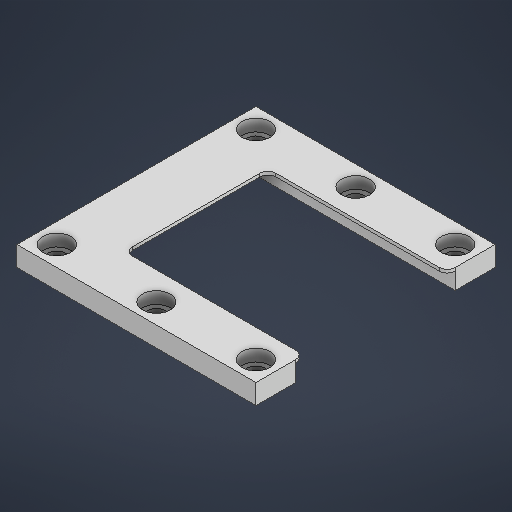
# Autodesk Inventor part: Flex Circuit Clamp V1
Saved by Autodesk Inventor 2026.2 (Build 302298010, 298A)
## iProperties
Created: 2026-05-04
Part Number: Flex Circuit Clamp V1
Material: Generic
Document SubType Name: Modeling
Designer: cfang
Density: 1 g/cm^3
Appearance: Default
Author: cfang
Autodesk Inventor part; units mm, degrees
ref_plane "YZ Plane" through (0, 0, 0) normal (1, 0, 0) x (0, 1, 0)
ref_plane "XZ Plane" through (0, 0, 0) normal (0, 1, 0) x (-1, 0, 0)
ref_plane "XY Plane" through (0, 0, 0) normal (0, 0, 1) x (1, 0, 0)
sketch "Sketch1" plane through (0, 0, 0) normal (0, 1, 0) x (-1, 0, 0)
  line L0 (-15, -15) -> (15, -15)
  line L1 (15, -15) -> (15, 15)
  line L2 (15, 15) -> (-15, 15)
  line L3 (-15, 15) -> (-15, -15)
  line L4 (-15, -15) -> (15, 15) construction
  line L5 (15, -15) -> (-15, 15) construction
  point P0 (0, 0)
  dimension "d0" = 30
  dimension "d1" = 30
  constraints: 12 end point, 2 midpoint, 2 parallel, 1 horizontal, 1 perpendicular
  measures "d0" distance of L0.end L1.end
  measures "d1" distance of L1.end L2.end
extrude "Extrusion1" add sketch "Sketch1" along normal blind 2.5
sketch "Sketch2" plane through (0, 2.5, 0) normal (0, 1, 0) x (1, 0, 0)
  line L0 (15, -15) -> (15, 15) projected
  line L1 (15, -10) -> (-10, -10)
  line L2 (-10, -10) -> (-10, 10)
  line L3 (-10, 10) -> (15, 10)
  line L4 (15, 10) -> (15, -10)
  point P0 (0, 0)
  point P1 (15, 10)
  dimension "d4" = 20
  dimension "d5" = 10
  dimension "d6" = 25
  constraints: 8 end point, 2 parallel, 1 horizontal, 1 perpendicular, 1 point on line
  measures "d4" distance of L1.end L2.end
  measures "d5" distance from line of L1 point (0, 0)
  measures "d6" distance of L1.start L1.end
extrude "Extrusion2" cut sketch "Sketch2" against normal through all
sketch "Sketch3" plane through (0, 2.5, 0) normal (0, 1, 0) x (1, 0, 0)
  line L0 (15, -10) -> (-10, -10) projected
  line L1 (-10, -10) -> (-10, 10) projected
  line L2 (-10, 10) -> (15, 10) projected
  line L3 (15, -10) -> (-10, -10)
  line L4 (-10, -10) -> (-10, -9)
  line L5 (-6.5, -9) -> (14, -9)
  line L6 (15, -10) -> (15, -10)
  line L7 (15, 10) -> (-10, 10)
  line L8 (-10, 10) -> (-10, 9)
  line L9 (-6.5, 9) -> (14, 9)
  line L10 (15, 10) -> (15, 10)
  line L11 (-10, -10) -> (-7.5, -10)
  line L12 (-7.5, -8) -> (-7.5, 8)
  line L13 (-7.5, 10) -> (-10, 10)
  line L14 (-10, 10) -> (-10, -10)
  arc A0 (15, -10) -> (14, -9) centre (14, -10) ccw
  arc A1 (-7.5, -8) -> (-6.5, -9) centre (-6.5, -8) ccw
  arc A2 (-6.5, 9) -> (-7.5, 8) centre (-6.5, 8) ccw
  arc A3 (14, 9) -> (15, 10) centre (14, 10) ccw
  point P0 (0, 0)
  point P1 (15, -9)
  point P2 (15, 9)
  point P3 (-7.5, -9)
  point P4 (-7.5, 9)
  dimension "d9" = 1
  dimension "d10" = 1
  dimension "d11" = 2.5
  dimension "d14" = 1
  constraints: 24 end point, 11 point on line, 8 point on circle, 8 tangent, 6 parallel, 4 centre point, 3 equal radius, 3 horizontal, 3 perpendicular
  measures "d9" distance between parallel lines of L0 L5
  measures "d10" distance between parallel lines of L2 L9
  measures "d11" distance between parallel lines of L1 L12
  measures "d14" radius of A0
extrude "Extrusion3" add sketch "Sketch3" against normal blind 0.4
sketch "Sketch4" plane through (0, 2.5, 0) normal (0, 1, 0) x (1, 0, 0)
  point P0 (0, 0)
  point P1 (12.5, -12.5)
  point P2 (-12.5, -12.5)
  point P3 (-12.5, 12.5)
  point P4 (12.5, 12.5)
  point P5 (-12.5, 0)
  point P6 (0, -12.5)
  point P7 (0, 12.5)
  dimension "d15" = 25
  dimension "d16" = 25
  dimension "d17" = 12.5
  dimension "d18" = 12.5
  constraints: 5 horizontal alignment, 5 vertical alignment
  measures "d15" distance of point (-12.5, 12.5) point (-12.5, -12.5)
  measures "d16" distance of point (-12.5, -12.5) point (12.5, -12.5)
  measures "d17" horizontal distance of point (-12.5, -12.5) point (0, 0)
  measures "d18" horizontal distance of point (-12.5, -12.5) point (0, 0)
hole "Hole1" at (12.5, 2.5, 12.5) at (-12.5, 2.5, 12.5) at (-12.5, 2.5, -12.5) at (12.5, 2.5, -12.5) at (0, 2.5, 12.5) at (0, 2.5, -12.5) direction (0, -1, 0) diameter 2.25 end through all counterbore diameter 3.5 counterbore depth 1.5
equation "\"d5\" = 0.5 * d4"
equation "\"d10\" = d9"
equation "\"d17\" = 0.5 * d15"
equation "\"d18\" = 0.5 * d16"
body "Solid1"
